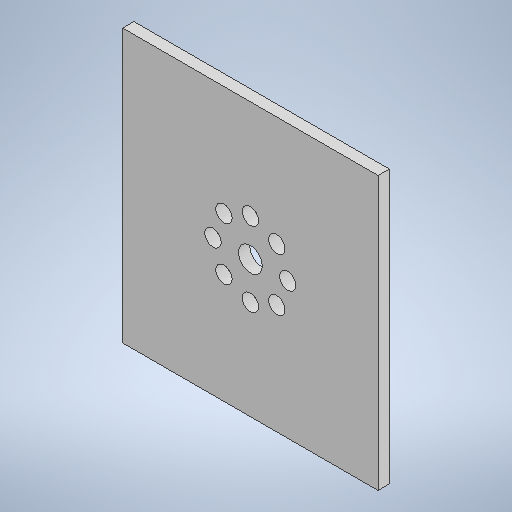
# Autodesk Inventor part: kosi_sita
Saved by Autodesk Inventor 2025.1 (Build 291241000, 241)
## iProperties
Created: 2024-08-31
Part Number: kosi_sita
Material: 一般
Document SubType Name: Modeling
Designer: right
Density: 1 g/cm^3
Appearance: 既定
Author: right
Autodesk Inventor part; units mm, degrees
ref_plane "YZ Plane" through (0, 0, 0) normal (1, 0, 0) x (0, 1, 0)
ref_plane "XZ Plane" through (0, 0, 0) normal (0, 1, 0) x (-1, 0, 0)
ref_plane "XY Plane" through (0, 0, 0) normal (0, 0, 1) x (1, 0, 0)
sketch "スケッチ1" plane through (0, 0, 0) normal (0, 0, 1) x (1, 0, 0)
  circle A0 centre (0, 0) radius 1.6
  circle A1 centre (0, 0) radius 5 construction
  circle A2 centre (0, 5) radius 1.1
  circle A3 centre (-3.5355, 3.5355) radius 1.1
  circle A4 centre (-5, 0) radius 1.1
  circle A5 centre (-3.5355, -3.5355) radius 1.1
  circle A6 centre (0, -5) radius 1.1
  circle A7 centre (3.5355, -3.5355) radius 1.1
  circle A8 centre (5, 0) radius 1.1
  circle A9 centre (3.5355, 3.5355) radius 1.1
  line L0 (-17.0862, -18.25) -> (17.0862, -18.25)
  line L1 (17.0862, -18.25) -> (17.0862, 18.25)
  line L2 (17.0862, 18.25) -> (-17.0862, 18.25)
  line L3 (-17.0862, 18.25) -> (-17.0862, -18.25)
  line L4 (-17.0862, -18.25) -> (17.0862, 18.25) construction
  line L5 (17.0862, -18.25) -> (-17.0862, 18.25) construction
  circle A10 centre (0, 0) radius 25
  line L6 (17.0862, 0) -> (-17.0862, 0) construction
  line L7 (-5, -18.25) -> (5, -18.25)
  line L8 (0, 18.25) -> (0, 0) construction
  dimension "d1" = 10
  dimension "d11" = 50
  dimension "d0" = 3.2
  dimension "d2" = 2.2
  dimension "d5" = 360
  dimension "d18" = 36.5
  dimension "d19" = 34.1724
  constraints: 18 end point, 9 centre point, 5 midpoint, 3 coincident, 3 vertical alignment, 2 parallel, 1 horizontal, 1 perpendicular, 22 other
  measures "d0" diameter of A0
  measures "d2" diameter of A2
  measures "d18" distance from line of L7.start L2
  measures "d19" distance of L1.end L2.end
extrude "押し出し1" add sketch "スケッチ1" along normal blind 1.5 contours L3 L2 L1 L0
